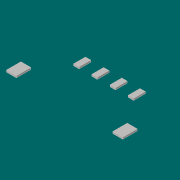
# Autodesk Inventor part: FH33-4S-1SH Land Pattren
Saved by Autodesk Inventor 2016 (Build 200138000, 138)
## iProperties
Created: 2015-08-26
Part Number: FH33-4S-1SH Land Pattren
Material: Generic
Document SubType Name: Modeling
Designer: Cosmic
Density: 1 g/cm^3
Appearance: Default
Author: Cosmic
Autodesk Inventor part; units mm, degrees
ref_plane "YZ Plane" through (0, 0, 0) normal (1, 0, 0) x (0, 1, 0)
ref_plane "XZ Plane" through (0, 0, 0) normal (0, 1, 0) x (-1, 0, 0)
ref_plane "XY Plane" through (0, 0, 0) normal (0, 0, 1) x (1, 0, 0)
sketch "Sketch1" plane through (0, 0, 0) normal (0, 0, 1) x (1, 0, 0)
  line L0 (-1.65, 2.65) -> (-1.35, 2.65)
  line L1 (-1.35, 2.65) -> (-1.35, 2)
  line L2 (-1.35, 2) -> (-1.65, 2)
  line L3 (-1.65, 2) -> (-1.65, 2.65)
  line L4 (-0.65, 2.65) -> (-0.35, 2.65)
  line L5 (-0.35, 2.65) -> (-0.35, 2)
  line L6 (-0.35, 2) -> (-0.65, 2)
  line L7 (-0.65, 2) -> (-0.65, 2.65)
  line L8 (0.35, 2.65) -> (0.65, 2.65)
  line L9 (0.65, 2.65) -> (0.65, 2)
  line L10 (0.65, 2) -> (0.35, 2)
  line L11 (0.35, 2) -> (0.35, 2.65)
  line L12 (1.35, 2.65) -> (1.65, 2.65)
  line L13 (1.65, 2.65) -> (1.65, 2)
  line L14 (1.65, 2) -> (1.35, 2)
  line L15 (1.35, 2) -> (1.35, 2.65)
  line L16 (-1.5, 2) -> (-1.5, 2.65)
  line L17 (-1.65, 2.325) -> (-1.35, 2.325)
  line L18 (-0.65, 2.325) -> (-0.35, 2.325)
  line L19 (-0.5, 2) -> (-0.5, 2.65)
  line L20 (0.5, 2) -> (0.5, 2.65)
  line L21 (0.35, 2.325) -> (0.65, 2.325)
  line L22 (1.5, 2.65) -> (1.5, 2)
  line L23 (1.35, 2.325) -> (1.65, 2.325)
  line L24 (-3.2, 0.65) -> (-2.65, 0.65)
  line L25 (-2.65, 0.65) -> (-2.65, -0.15)
  line L26 (-2.65, -0.15) -> (-3.2, -0.15)
  line L27 (-3.2, -0.15) -> (-3.2, 0.65)
  line L28 (2.65, 0.65) -> (3.2, 0.65)
  line L29 (3.2, 0.65) -> (3.2, -0.15)
  line L30 (3.2, -0.15) -> (2.65, -0.15)
  line L31 (2.65, -0.15) -> (2.65, 0.65)
  line L32 (-2.925, 0.65) -> (-2.925, -0.15)
  line L33 (-3.2, 0.25) -> (-2.65, 0.25)
  line L34 (2.925, -0.15) -> (2.925, 0.65)
  line L35 (2.65, 0.25) -> (3.2, 0.25)
  line L36 (3.25, 2.15) -> (3.25, 0.5)
  line L37 (3.25, 0.5) -> (3, 0.5)
  line L38 (3, 0.5) -> (3, 0)
  line L39 (3, 0) -> (-3, 0)
  line L40 (-3, 0) -> (-3, 0.5)
  line L41 (-3, 0.5) -> (-3.25, 0.5)
  line L42 (-3.25, 0.5) -> (-3.25, 2.15)
  line L43 (-3.25, 2.15) -> (3.25, 2.15)
  line L44 (0, 0) -> (0, 2.15)
  dimension "d2" = 0.3
  dimension "d3" = 0.65
  dimension "d4" = 0.3
  dimension "d5" = 0.65
  dimension "d6" = 0.3
  dimension "d7" = 0.65
  dimension "d8" = 0.3
  dimension "d9" = 0.65
  dimension "d10" = 1
  dimension "d11" = 1
  dimension "d12" = 1
  dimension "d13" = 0.8
  dimension "d14" = 0.55
  dimension "d15" = 0.55
  dimension "d16" = 0.8
  dimension "d17" = 5.3
  dimension "d18" = 6.5
  dimension "d19" = 2.8
  dimension "d20" = 2.65
  dimension "d22" = 0.15
  dimension "d23" = 0.2
  dimension "d24" = 2.15
  dimension "d25" = 0.15
  dimension "d28" = 0.5
  constraints: 90 end point, 26 midpoint, 12 parallel, 11 perpendicular, 7 horizontal, 3 collinear, 3 point on line, 1 coincident, 1 vertical
  measures "d2" distance of L1.end L2.end
  measures "d3" distance of L0.end L1.end
  measures "d4" distance of L5.end L6.end
  measures "d5" distance of L4.end L5.end
  measures "d6" distance of L9.end L10.end
  measures "d7" distance of L8.end L9.end
  measures "d8" distance of L13.end L14.end
  measures "d9" distance of L12.end L13.end
  measures "d10" distance between parallel lines of L20 L22
  measures "d11" distance between parallel lines of L19 L20
  measures "d12" distance between parallel lines of L16 L19
  measures "d13" distance of L28.end L29.end
  measures "d14" distance of L29.end L30.end
  measures "d15" distance of L25.end L26.end
  measures "d16" distance of L26.end L24.start
  measures "d17" distance between parallel lines of L31 L25
  measures "d18" distance between parallel lines of L42 L36
  measures "d19" distance between parallel lines of L26 L0
  measures "d20" distance from line of point (0, 0) L31
  measures "d22" distance between parallel lines of L37 L28
  measures "d23" distance between parallel lines of L29 L38
  measures "d24" distance between parallel lines of L43 L39
  measures "d25" distance between parallel lines of L26 L39
  measures "d28" distance from line of L44.end L19
extrude "Extrusion1" add sketch "Sketch1" along normal blind 0.1 contours L0 L16 L17 L3 | L0 L1 L17 L16 | L17 L16 L43 L3 | L17 L1 L43 L16 | L43 L16 L2 L3 | L43 L1 L2 L16 | L43 L19 L6 L7 | L7 L18 L19 L43 | L41 L40 L33 L27 | L27 L24 L32 L33 L40 L41 | L7 L4 L19 L18 | L43 L5 L6 L19 | L19 L18 L5 L43 | L33 L40 L39 L32 L26 L27 | L19 L4 L5 L18 | L33 L32 L39 L40 | L24 L25 L33 L32 | L32 L39 L25 L26 | L33 L25 L39 L32 | L43 L20 L10 L11 | L11 L21 L20 L43 | L11 L8 L20 L21 | L43 L9 L10 L20 | L20 L21 L9 L43 | L39 L34 L30 L31 | L31 L35 L34 L39 | L20 L8 L9 L21 | L31 L28 L34 L35 | L39 L38 L35 L29 L30 L34 | L34 L35 L38 L39 | L43 L22 L14 L15 | L15 L23 L22 L43 | L34 L28 L29 L37 L38 L35 | L15 L12 L22 L23 | L43 L13 L14 L22 | L22 L23 L13 L43 | L38 L37 L29 L35 | L22 L12 L13 L23
equation "\"d15\" = d14"
equation "\"d16\" = d13"
equation "\"d20\" = 0.5 * d17"
equation "\"d28\" = 0.5 * d11"
body "Solid1"
